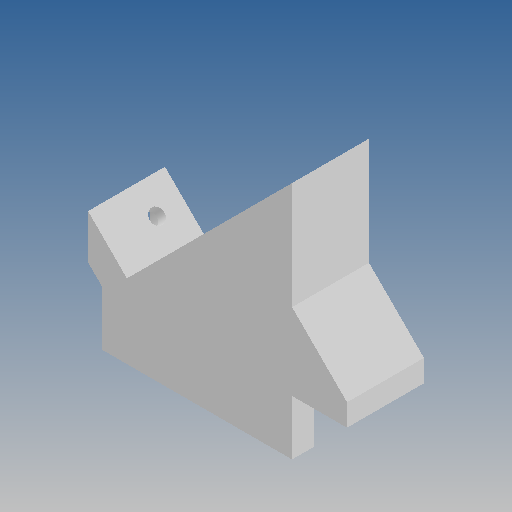
# Autodesk Inventor part: Print_Parts_L1
Saved by Autodesk Inventor 2020 (Build 240168000, 168)
## iProperties
Created: 2020-11-09
Part Number: Print_Parts_L1
Material: 一般
Document SubType Name: Modeling
Designer: kenta iguchi
Density: 1 g/cm^3
Appearance: 既定
Author: kenta iguchi
Autodesk Inventor part; units mm, degrees
ref_plane "YZ Plane" through (0, 0, 0) normal (1, 0, 0) x (0, 1, 0)
sketch "スケッチ1" plane through (0, 0, 0) normal (0, 0, 1) x (1, 0, 0)
  line L0 (0, 0) -> (8, 0)
  line L1 (8, 0) -> (8, 7)
  line L2 (8, 7) -> (0, 7)
  line L3 (0, 7) -> (0, 0)
  line L4 (8, 7) -> (68.1041, 67.1041)
  line L5 (68.1041, 67.1041) -> (68.1041, 0)
  line L6 (68.1041, 0) -> (-2.6124, 0)
  dimension "d0" = 8
  dimension "d1" = 7
  dimension "d3" = 85
  dimension "d245" = 45
  constraints: 14 end point, 2 horizontal alignment, 2 parallel, 1 horizontal, 1 perpendicular, 1 vertical
  measures "d0" distance between parallel lines of L1 L3
  measures "d1" distance of L0.end L1.end
  measures "d3" distance of L1.end L4.end
  measures "d245" angle of L4 L6
extrude "押し出し1" add sketch "スケッチ1" along normal blind 20
sketch "スケッチ15" plane through (0, 0, 20) normal (0, 0, 1) x (1, 0, 0)
  line L0 (68.1041, 67.1041) -> (8, 7) projected
  line L1 (8, 7) -> (0, 7) projected
  line L2 (0, 7) -> (0, 0) projected
  line L3 (8, 7) -> (-6.1421, 21.1421)
  line L4 (-6.1421, 21.1421) -> (-6.1421, 0)
  line L5 (-6.1421, 0) -> (0, 0)
  dimension "d92" = 20
  constraints: 6 end point, 2 perpendicular, 1 parallel
  measures "d92" distance of L0.end L3.end
extrude "押し出し10" add sketch "スケッチ15" against normal up to surface (20 mm away)
chamfer "面取り7" distance 5 angle 45 1 edges at (-6.1421, 0, 10)
sketch "スケッチ16" plane through (-6.1421, 21.1421, 20) normal (0.7071068, 0.7071068, 0) x (0, 0, -1)
  point P0 (20, -19.2929)
  point P1 (10, -10)
hole "穴6" at (0.9289, 14.0711, 10) direction (-0.7071068, -0.7071068, 0) diameter 5.3 depth 58
ref_plane "作業平面2" through (-8.9706, 18.3137, 20) normal (0.7071068, 0.7071068, 0) x (0, 0, -1)
sketch "スケッチ17" plane through (-8.9706, 18.3137, 20) normal (0.7071068, 0.7071068, 0) x (0, 0, -1)
  arc A0 (12.2411, -11.4142) -> (7.7589, -11.4142) centre (10, -10) ccw projected
  point P0 (20, -19.2929)
hole "穴7" at (-1.8995, 11.2426, 10) direction (-0.7071068, -0.7071068, 0) diameter 9.5 depth 58
sketch "スケッチ18" plane through (68.1041, 67.1041, 20) normal (-0.7071068, 0.7071068, 0) x (0.7071068, 0.7071068, 0)
  line L0 (0, 20) -> (-85, 20) projected
  line L1 (-85, 20) -> (-85, 0) projected
  line L2 (0, 20) -> (0, 0) projected
  point P0 (-95.6066, 20)
  point P1 (-75, 10)
  point P2 (-42.5, 10)
  point P3 (-10, 10)
  dimension "d119" = 10
  dimension "d120" = 10
  dimension "d121" = 10
  dimension "d122" = 32.5
  constraints: 2 horizontal alignment
  measures "d119" distance from line of L0 point (-75, 10)
  measures "d120" distance from line of point (-75, 10) L1
  measures "d121" distance from line of L2 point (-10, 10)
  measures "d122" distance of point (-42.5, 10) point (-75, 10)
hole "穴8" [suppressed]
ref_plane "作業平面3" through (72.3467, 62.8614, 20) normal (-0.7071068, 0.7071068, 0) x (0.7071068, 0.7071068, 0)
sketch "スケッチ19" plane through (72.3467, 62.8614, 20) normal (-0.7071068, 0.7071068, 0) x (0.7071068, 0.7071068, 0)
  line L0 (0, 20) -> (-85, 20) projected
  line L1 (-85, 20) -> (-85, 0) projected
  line L2 (0, 0) -> (-85, 0) projected
  line L3 (0, 20) -> (0, 0) projected
  point P0 (-95.6066, 20)
hole "穴9" [suppressed]
sketch "スケッチ20" plane through (0, 0, 20) normal (0, 0, 1) x (1, 0, 0)
  line L0 (68.1041, 0) -> (68.1041, 67.1041) projected
  line L1 (68.1041, 67.1041) -> (8, 7) projected
  line L2 (-6.1421, 21.1421) -> (-6.1421, 0) projected
  line L3 (68.1041, 67.1041) -> (8, 7)
  line L4 (8, 7) -> (-6.1421, 21.1421)
  line L5 (-6.1421, 21.1421) -> (53.9619, 81.2462)
  line L6 (53.9619, 81.2462) -> (68.1041, 67.1041)
  line L7 (-5.2583, 14.6014) -> (1.4593, 7.8839) projected
  line L8 (-1.1421, 0) -> (-6.1421, 5) projected
  line L9 (-1.1421, 0) -> (68.1041, 0) projected
  line L10 (68.1041, 0) -> (68.1041, 67.1041) projected
  line L11 (68.1041, 67.1041) -> (8, 7) projected
  line L12 (8, 7) -> (-6.1421, 21.1421) projected
  line L13 (-6.1421, 21.1421) -> (-6.1421, 5) projected
  point P0 (-3.4715, 23.383)
  point P1 (-3.4715, 23.383)
  point P2 (-6.1421, 0)
  constraints: 8 end point, 3 equal length, 1 perpendicular, 1 other
extrude "押し出し11" add sketch "スケッチ20" along normal blind 8 contours L9 L8 L2 L4 L1 L0
sketch "スケッチ21" plane through (0, 0, 28) normal (0, 0, 1) x (1, 0, 0)
  line L0 (68.1041, 67.1041) -> (8, 7) projected
  line L1 (8, 7) -> (-6.1421, 21.1421) projected
  line L2 (-6.1421, 21.1421) -> (-6.1421, 5) projected
  line L3 (-6.1421, 5) -> (-1.1421, 0) projected
  line L4 (-1.1421, 0) -> (68.1041, 0) projected
  line L5 (68.1041, 0) -> (68.1041, 67.1041) projected
  line L6 (-1.1421, 0) -> (68.1041, 0)
  line L7 (68.1041, 0) -> (68.1041, -20)
  line L8 (68.1041, -20) -> (-1.1421, -20)
  line L9 (-1.1421, -20) -> (-1.1421, 0)
  dimension "d247" = 20
  constraints: 8 end point, 2 parallel, 1 horizontal, 1 perpendicular, 1 vertical alignment
  measures "d247" distance of L6.end L7.end
extrude "押し出し12" add sketch "スケッチ21" against normal blind 8 contours L7 L8 L9 L4
sketch "スケッチ23" plane through (68.1041, 0, 0) normal (1, 0, 0) x (0, 0, -1)
  line L0 (0, 0) -> (0, 67.1041) projected
  line L1 (0, 0) -> (-20, 0)
  line L2 (0, 0) -> (-28, 0)
  line L3 (-28, 0) -> (-28, 8)
  line L4 (-28, 8) -> (0, 8)
  line L5 (0, 8) -> (0, 0)
  point P0 (-28, 55.754)
  point P1 (0, 8)
  constraints: 10 end point, 2 parallel, 1 horizontal, 1 perpendicular
extrude "押し出し13" add sketch "スケッチ23" along normal blind 20
chamfer "面取り8" distance 20 angle 45 1 edges at (68.1041, 8, 14)
sketch "スケッチ24" plane through (1.5285, 0, 20) normal (0, -1, 0) x (1, 0, 0)
  line L0 (96.0995, -20) -> (0, -20) projected
  line L1 (96.0995, 8) -> (96.0995, -20) projected
  point P0 (-1.5285, -20)
  point P1 (86.0995, -10)
  dimension "d161" = 10
  dimension "d162" = 10
  measures "d161" distance from line of L1 point (86.099, -10)
  measures "d162" distance from line of L0 point (86.099, -10)
hole "穴11" [suppressed]
sketch "スケッチ25" plane through (1.5285, 6, 20) normal (0, -1, 0) x (1, 0, 0)
  circle A0 centre (86.0995, -10) radius 2.15 projected
  point P0 (-1.5285, -20)
sketch "スケッチ27" plane through (0, 0, 28) normal (0, 0, 1) x (1, 0, 0)
  line L0 (68.1041, -20) -> (68.1041, 0) projected
  line L1 (77.6279, 0) -> (97.6279, 0) projected
  line L2 (77.6279, -20) -> (1.5285, -20) projected
  line L3 (97.6279, 0) -> (1.5285, 0) projected
  line L4 (77.6279, -20) -> (97.6279, -20)
  line L5 (97.6279, -20) -> (97.6279, 0)
  line L6 (97.6279, 0) -> (77.6279, 0)
  line L7 (77.6279, 0) -> (77.6279, -20)
  point P0 (0, 0)
  constraints: 8 end point, 2 parallel, 1 horizontal, 1 perpendicular
sketch "スケッチ22" plane through (0, 0, 28) normal (0, 0, 1) x (1, 0, 0)
  line L0 (1.5285, 0) -> (1.5285, -20) projected
  line L1 (1.5285, -20) -> (77.6279, -20) projected
  line L2 (97.6279, 8) -> (97.6279, -20) projected
  point P0 (0, 0)
  point P1 (11.5285, -10)
  point P2 (36.895, -10)
  point P3 (62.2614, -10)
  point P4 (87.6279, -10)
  dimension "d143" = 10
  dimension "d144" = 10
  dimension "d185" = 10
  dimension "d186" = 76.0995
  dimension "d187" = 25.3665
  dimension "d188" = 25.3665
  constraints: 3 horizontal alignment
  measures "d143" distance from line of point (11.528, -10) L1
  measures "d144" distance from line of point (11.528, -10) L0
  measures "d185" distance from line of L2 point (87.628, -10)
  measures "d186" distance of point (87.628, -10) point (11.528, -10)
  measures "d187" distance of point (36.895, -10) point (11.528, -10)
  measures "d188" distance of point (62.261, -10) point (36.895, -10)
sketch "スケッチ28" plane through (0, 0, 20) normal (0, 0, -1) x (-1, 0, 0)
  line L0 (-77.6279, 55.754) -> (-71.9329, 63.8873) projected
  line L1 (-77.6279, 55.754) -> (-8, 7) projected
  line L2 (-8, 7) -> (3.4715, 23.383) projected
  line L3 (-2.2642, 15.1915) -> (-101.3499, 84.572)
  line L4 (-68.1041, 67.1041) -> (-8, 7) projected
  line L5 (-39.5723, 38.5723) -> (-36.5318, 35.5318) projected
  line L6 (-16.5913, 15.5913) -> (-13.5508, 12.5508) projected
  line L7 (-62.5533, 61.5533) -> (-59.5127, 58.5127) projected
  line L8 (-70.2375, 50.5791) -> (-66.7686, 48.1502) projected
  line L9 (-68.1041, 67.1041) -> (-8, 7) projected
  point P0 (0, 0)
  point P1 (-10.4558, 20.9273)
  point P2 (-37.0782, 39.5685)
  point P3 (-63.7006, 58.2098)
  dimension "d196" = 10
  dimension "d197" = 32.5
  dimension "d198" = 65
  constraints: 3 point on line, 2 end point, 1 midpoint, 1 parallel
  measures "d196" distance from line of point (-63.701, 58.21) L0
  measures "d197" distance of point (-37.078, 39.569) point (-63.701, 58.21)
  measures "d198" distance of point (-10.456, 20.927) point (-63.701, 58.21)
sketch "スケッチ29" plane through (0, 0, 28) normal (0, 0, 1) x (1, 0, 0)
  circle A0 centre (37.0782, 39.5685) radius 2.15 projected
  circle A1 centre (10.4558, 20.9273) radius 2.15 projected
  circle A2 centre (63.7006, 58.2098) radius 2.15 projected
  point P0 (0, 0)
sketch "スケッチ30" plane through (0, 0, 28) normal (0, 0, 1) x (1, 0, 0)
  circle A0 centre (10.4558, 20.9273) radius 4 projected
  point P0 (0, 0)
sketch "スケッチ31" plane through (1.5285, 0, 0) normal (0, -1, 0) x (1, 0, 0)
  ellipse E0 centre (23.5807, 10) end of major axis (28.4638, 10) minor radius 4 projected
  ellipse E1 centre (63.2559, 10) end of major axis (68.139, 10) minor radius 4 projected
  circle A0 centre (86.0995, 10) radius 2.15 projected
  line L0 (96.0995, 20) -> (96.0995, 0) projected
  line L1 (0, 0) -> (0, 20) projected
  line L2 (96.0995, 7.1) -> (0, 7.1)
  line L3 (0, 7.1) -> (0, 12.9)
  line L4 (0, 12.9) -> (96.0995, 12.9)
  line L5 (96.0995, 12.9) -> (96.0995, 7.1)
  line L6 (51.228, 7.1) -> (36.228, 7.1)
  line L7 (36.228, 7.1) -> (36.228, 12.9)
  line L8 (36.228, 12.9) -> (51.228, 12.9)
  line L9 (51.228, 12.9) -> (51.228, 7.1)
  line L10 (9.7875, 12.9) -> (0, 12.9)
  line L11 (0, 12.9) -> (0, 7.1)
  line L12 (0, 7.1) -> (9.7875, 7.1)
  line L13 (9.7875, 7.1) -> (9.7875, 12.9)
  line L14 (76.0995, 7.1) -> (71.0995, 7.1)
  line L15 (71.0995, 7.1) -> (71.0995, 12.9)
  line L16 (71.0995, 12.9) -> (76.0995, 12.9)
  line L17 (76.0995, 12.9) -> (76.0995, 7.1)
  point P0 (96.0995, 2)
  point P1 (-1.5285, 0)
  point P2 (0, 7.1)
  point P3 (20.2175, 7.1)
  point P4 (20.2175, 12.9)
  point P5 (59.8927, 7.1)
  point P6 (59.8927, 12.9)
  point P7 (26.944, 12.9)
  point P8 (26.944, 7.1)
  point P9 (76.0995, 12.9)
  point P10 (66.6191, 12.9)
  point P11 (66.6191, 7.1)
  dimension "d220" = 5.8
  dimension "d221" = 2.9
  dimension "d223" = 15
  dimension "d224" = 10
  constraints: 32 end point, 8 parallel, 7 point on line, 4 horizontal, 4 perpendicular, 2 other
  measures "d220" distance between parallel lines of L2 L4
  measures "d221" distance from line of L2 A0.centre
  measures "d223" distance between parallel lines of L7 L9
  measures "d224" distance from line of L17 A0.centre
sketch "スケッチ33" plane through (42.2947, 32.8094, 10) normal (0.7071068, -0.7071068, 0) x (0, 0, 1)
  circle A0 centre (0, 0) radius 4 projected
  circle A1 centre (0, 32.5) radius 2.15 projected
  circle A2 centre (0, 32.5) radius 4 projected
  point P0 (-10, 53.1066)
sketch "スケッチ34" plane through (87.6279, -10, 24) normal (0, 0, 1) x (1, 0, 0)
  circle A0 centre (0, 0) radius 2.15 projected
  circle A1 centre (-25.3665, 0) radius 4 projected
  circle A2 centre (-25.3665, 0) radius 2.15 projected
  circle A3 centre (-76.0995, 0) radius 2.15 projected
  circle A4 centre (-77.1722, 30.9273) radius 2.65 projected
  circle A5 centre (-50.5497, 49.5685) radius 2.15 projected
  circle A6 centre (-23.9273, 68.2098) radius 2.15 projected
  circle A7 centre (-23.9273, 68.2098) radius 4 projected
  line L0 (2.15, 2.15) -> (-2.15, 2.15)
  line L1 (-2.15, 2.15) -> (-2.15, -2.15)
  line L2 (-2.15, -2.15) -> (2.15, -2.15)
  line L3 (2.15, -2.15) -> (2.15, 2.15)
  line L4 (2.15, 2.15) -> (-2.15, -2.15) construction
  line L5 (-2.15, 2.15) -> (2.15, -2.15) construction
  line L6 (-23.2165, 2.15) -> (-27.5165, 2.15)
  line L7 (-27.5165, 2.15) -> (-27.5165, -2.15)
  line L8 (-27.5165, -2.15) -> (-23.2165, -2.15)
  line L9 (-23.2165, -2.15) -> (-23.2165, 2.15)
  line L10 (-23.2165, 2.15) -> (-27.5165, -2.15) construction
  line L11 (-27.5165, 2.15) -> (-23.2165, -2.15) construction
  line L12 (-73.9495, 2.15) -> (-78.2495, 2.15)
  line L13 (-78.2495, 2.15) -> (-78.2495, -2.15)
  line L14 (-78.2495, -2.15) -> (-73.9495, -2.15)
  line L15 (-73.9495, -2.15) -> (-73.9495, 2.15)
  line L16 (-73.9495, 2.15) -> (-78.2495, -2.15) construction
  line L17 (-78.2495, 2.15) -> (-73.9495, -2.15) construction
  line L18 (-74.5222, 33.5773) -> (-79.8222, 33.5773)
  line L19 (-79.8222, 33.5773) -> (-79.8222, 28.2773)
  line L20 (-79.8222, 28.2773) -> (-74.5222, 28.2773)
  line L21 (-74.5222, 28.2773) -> (-74.5222, 33.5773)
  line L22 (-74.5222, 33.5773) -> (-79.8222, 28.2773) construction
  line L23 (-79.8222, 33.5773) -> (-74.5222, 28.2773) construction
  line L24 (-48.3997, 51.7185) -> (-52.6997, 51.7185)
  line L25 (-52.6997, 51.7185) -> (-52.6997, 47.4185)
  line L26 (-52.6997, 47.4185) -> (-48.3997, 47.4185)
  line L27 (-48.3997, 47.4185) -> (-48.3997, 51.7185)
  line L28 (-48.3997, 51.7185) -> (-52.6997, 47.4185) construction
  line L29 (-52.6997, 51.7185) -> (-48.3997, 47.4185) construction
  line L30 (-21.7773, 70.3598) -> (-26.0773, 70.3598)
  line L31 (-26.0773, 70.3598) -> (-26.0773, 66.0598)
  line L32 (-26.0773, 66.0598) -> (-21.7773, 66.0598)
  line L33 (-21.7773, 66.0598) -> (-21.7773, 70.3598)
  line L34 (-21.7773, 70.3598) -> (-26.0773, 66.0598) construction
  line L35 (-26.0773, 70.3598) -> (-21.7773, 66.0598) construction
  circle A8 centre (-23.9273, 68.2098) radius 2.15 projected
  circle A9 centre (-50.733, 0) radius 2.15 projected
  line L36 (-52.883, 2.15) -> (-48.583, 2.15)
  line L37 (-48.583, 2.15) -> (-48.583, -2.15)
  line L38 (-48.583, -2.15) -> (-52.883, -2.15)
  line L39 (-52.883, -2.15) -> (-52.883, 2.15)
  line L40 (-52.883, 2.15) -> (-48.583, -2.15) construction
  line L41 (-48.583, 2.15) -> (-52.883, -2.15) construction
  point P0 (-87.6279, 10)
  constraints: 84 end point, 14 midpoint, 14 parallel, 14 tangent, 7 horizontal, 7 perpendicular, 1 point on line
sketch "スケッチ35" plane through (87.6279, -10, 24) normal (0, 0, 1) x (1, 0, 0)
  line L0 (2.15, -2.15) -> (-2.15, -2.15) projected
  line L1 (-2.15, 2.15) -> (2.15, 2.15) projected
  circle A0 centre (0, 0) radius 4 projected
  line L2 (-23.2165, 2.15) -> (-23.2165, -2.15) projected
  line L3 (-23.2165, -2.15) -> (-27.5165, -2.15) projected
  line L4 (-27.5165, -2.15) -> (-27.5165, 2.15) projected
  line L5 (-27.5165, 2.15) -> (-23.2165, 2.15) projected
  circle A1 centre (-25.3665, 0) radius 4 projected
  line L6 (-52.883, 2.15) -> (-48.583, 2.15) projected
  line L7 (-48.583, 2.15) -> (-48.583, -2.15) projected
  line L8 (-48.583, -2.15) -> (-52.883, -2.15) projected
  line L9 (-52.883, -2.15) -> (-52.883, 2.15) projected
  circle A2 centre (-50.733, 0) radius 4 projected
  line L10 (-78.2495, 2.15) -> (-73.9495, 2.15) projected
  line L11 (-73.9495, 2.15) -> (-73.9495, -2.15) projected
  line L12 (-73.9495, -2.15) -> (-78.2495, -2.15) projected
  line L13 (-78.2495, -2.15) -> (-78.2495, 2.15) projected
  circle A3 centre (-76.0995, 0) radius 4 projected
  circle A4 centre (-77.1722, 30.9273) radius 4.75 projected
  circle A5 centre (-50.5497, 49.5685) radius 4 projected
  circle A6 centre (-23.9273, 68.2098) radius 4 projected
  line L14 (18.1594, -2.15) -> (-105.0634, -2.15)
  line L15 (-105.0634, -2.15) -> (-105.0634, 2.15)
  line L16 (-105.0634, 2.15) -> (18.1594, 2.15)
  line L17 (18.1594, 2.15) -> (18.1594, -2.15)
  circle A7 centre (-23.9273, 68.2098) radius 4 projected
  line L18 (-21.7773, 71.5828) -> (-26.0773, 71.5828)
  line L19 (-26.0773, 71.5828) -> (-26.0773, 64.8367)
  line L20 (-26.0773, 64.8367) -> (-21.7773, 64.8367)
  line L21 (-21.7773, 64.8367) -> (-21.7773, 71.5828)
  line L22 (-21.7773, 71.5828) -> (-26.0773, 64.8367) construction
  line L23 (-26.0773, 71.5828) -> (-21.7773, 64.8367) construction
  circle A8 centre (-50.5497, 49.5685) radius 4 projected
  line L24 (-52.6997, 46.1955) -> (-48.3997, 46.1955)
  line L25 (-48.3997, 46.1955) -> (-48.3997, 52.9416)
  line L26 (-48.3997, 52.9416) -> (-52.6997, 52.9416)
  line L27 (-52.6997, 52.9416) -> (-52.6997, 46.1955)
  line L28 (-52.6997, 46.1955) -> (-48.3997, 52.9416) construction
  line L29 (-48.3997, 46.1955) -> (-52.6997, 52.9416) construction
  circle A9 centre (-77.1722, 30.9273) radius 4.75 projected
  line L30 (-74.5222, 34.8694) -> (-79.8222, 34.8694)
  line L31 (-79.8222, 34.8694) -> (-79.8222, 26.9852)
  line L32 (-79.8222, 26.9852) -> (-74.5222, 26.9852)
  line L33 (-74.5222, 26.9852) -> (-74.5222, 34.8694)
  line L34 (-74.5222, 34.8694) -> (-79.8222, 26.9852) construction
  line L35 (-79.8222, 34.8694) -> (-74.5222, 26.9852) construction
  point P0 (-87.6279, 10)
  point P1 (-3.3731, 2.15)
  point P2 (-3.3731, -2.15)
  point P3 (3.3731, -2.15)
  point P4 (3.3731, 2.15)
  point P5 (-28.7395, 2.15)
  point P6 (-28.7395, -2.15)
  point P7 (-21.9934, -2.15)
  point P8 (-21.9934, 2.15)
  point P9 (-54.106, 2.15)
  point P10 (-54.106, -2.15)
  point P11 (-47.3599, -2.15)
  point P12 (-47.3599, 2.15)
  point P13 (-72.7264, 2.15)
  point P14 (-79.4725, 2.15)
  point P15 (-79.4725, -2.15)
  point P16 (-72.7264, -2.15)
  point P17 (-48.3997, 52.9416)
  point P18 (-52.6997, 52.9416)
  point P19 (-21.7773, 71.5828)
  point P20 (-26.0773, 71.5828)
  constraints: 44 end point, 8 parallel, 6 midpoint, 4 horizontal, 4 perpendicular, 3 point on circle, 2 horizontal alignment
equation "\"d187\" = 0.333333 * d186"
equation "\"d188\" = d187"
